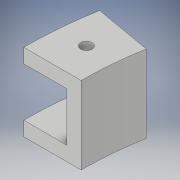
# Autodesk Inventor part: Inner_mount
Saved by Autodesk Inventor 2019 (Build 230136000, 136)
## iProperties
Created: 2019-05-19
Part Number: Inner_mount
Material: Generic
Document SubType Name: Modeling
Designer: Jorian Brusind
Density: 1 g/cm^3
Appearance: Default
Author: Jorian Brusind
Autodesk Inventor part; units mm, degrees
ref_plane "YZ Plane" through (0, 0, 0) normal (1, 0, 0) x (0, 1, 0)
ref_plane "XZ Plane" through (0, 0, 0) normal (0, 1, 0) x (-1, 0, 0)
ref_plane "XY Plane" through (0, 0, 0) normal (0, 0, 1) x (1, 0, 0)
sketch "Sketch1" plane through (0, 0, 0) normal (0, 1, 0) x (-1, 0, 0)
  line L0 (0, 0) -> (125, 0) construction
  line L1 (0, 0) -> (125, 0) construction
  line L2 (0, 0) -> (123.101, -21.706) construction
  line L3 (0, 0) -> (300, 0) construction
  line L4 (0, 0) -> (300, 0) construction
  line L5 (140, 0) -> (125, 0)
  line L6 (137.8731, -24.3107) -> (123.101, -21.706)
  line L7 (124.5243, -10.8945) -> (129.5053, -11.3302)
  circle A0 centre (129.5053, -11.3302) radius 2
  arc A1 (137.8731, -24.3107) -> (140, 0) centre (0, 0) ccw
  arc A2 (123.101, -21.706) -> (124.5243, -10.8945) centre (0, 0) ccw
  arc A3 (124.5243, -10.8945) -> (125, 0) centre (0, 0) ccw
  dimension "d1" = 0
  dimension "d2" = 10
  dimension "d4" = 0
  dimension "d7" = 5
  dimension "d8" = 5
  dimension "d9" = 4
  dimension "d28" = 140
  dimension "d29" = 125
  dimension "d31" = 14.7721
  constraints: 16 end point, 6 coincident, 6 point on circle, 4 centre point, 2 collinear, 2 horizontal, 1 point on line
  measures "d1" distance between parallel lines of L0 L1
  measures "d2" angle of L2 L0
  measures "d4" distance between parallel lines of L3 L4
  measures "d7" distance of L7.start L7.end
  measures "d8" angle of L0 L7
  measures "d9" diameter of A0
  measures "d28" radius of A1
  measures "d29" radius of A2
  measures "d31" horizontal distance of L6.start L2.end
extrude "Extrusion1" add sketch "Sketch1" along normal blind 5
sketch "Sketch3" plane through (0, 5, 0) normal (0, 1, 0) x (1, 0, 0)
  arc A0 (-123.101, 21.706) -> (-125, 0) centre (0, 0) ccw projected
  arc A1 (-123.101, 21.706) -> (-125, 0) centre (0, 0) ccw
  arc A2 (-118.1769, 20.8378) -> (-120, 0) centre (0, 0) ccw
  line L0 (0, 0) -> (-118.1769, 20.8378) construction
  line L1 (0, 0) -> (-120, 0) construction
  line L2 (-123.101, 21.706) -> (-118.1769, 20.8378)
  line L3 (-125, 0) -> (-120, 0)
  dimension "d33" = 120
  dimension "d34" = 10
  constraints: 8 end point, 4 point on circle, 2 centre point, 2 coincident, 1 horizontal
  measures "d33" radius of A2
  measures "d34" angle of L0 L1
extrude "Extrusion4" add sketch "Sketch3" along normal blind 27 from surface at -5
pattern_linear "Rectangular Pattern3" count 2 spacing 22 along (0, 1, 0) of "Extrusion1"
body "Solid1"
